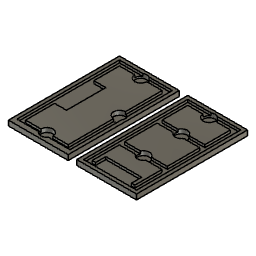
Circuit Template v1 v1 (Autodesk Fusion 360 design; units mm, degrees)
Autodesk Fusion 360 part; units mm, degrees
note: some values were not read from the file. Set by a fixed rule: which sketch regions a step uses.
sketch "Sketch1" plane through (0, 0, 0) normal (0, 0, 1) x (1, 0, 0)
  line L0 (0, 0) -> (88.9, 0)
  line L1 (88.9, 0) -> (88.9, 165.1)
  line L2 (88.9, 165.1) -> (0, 165.1)
  line L3 (0, 165.1) -> (0, 0)
  constraint horizontal L0
  constraint vertical L1
  constraint horizontal L2
  constraint vertical L3
  constraint coincident L0.start L3.end
extrude "Extrude1" add sketch "Sketch1" along normal blind 7.62 makes body 1
sketch "Sketch2" plane through (0, 0, 7.62) normal (0, 0, 1) x (-1, 0, 0)
  line L0 (0, -165.1) -> (0, 0)
  line L1 (0, 0) -> (-88.9, 0)
  line L2 (-88.9, 0) -> (-88.9, -165.1)
  line L3 (-88.9, -165.1) -> (0, -165.1)
  line L4 (-5.08, -7.62) -> (-83.82, -7.62)
  line L5 (-83.82, -7.62) -> (-83.82, -160.02)
  line L6 (-83.82, -160.02) -> (-5.08, -160.02)
  line L7 (-5.08, -160.02) -> (-5.08, -7.62)
  line L8 (-12.7, -152.4) -> (-76.2, -152.4)
  line L9 (-76.2, -152.4) -> (-76.2, -12.7)
  line L10 (-76.2, -12.7) -> (-12.7, -12.7)
  line L11 (-12.7, -12.7) -> (-12.7, -152.4)
  constraint horizontal L4
  constraint vertical L5
  constraint horizontal L6
  constraint vertical L7
  constraint horizontal L8
  constraint vertical L9
  constraint horizontal L10
  constraint vertical L11
copy_body "CopyPasteBodies1" bodies 1 makes body 2
move_body "Move1" bodies 2 to x (1, 0, 0) y (0, 1, 0) z (0, 0, 1) at (101.6, 0, 0)
sketch "Sketch3" plane through (0, 0, 7.62) normal (0, 0, 1) x (1, 0, 0)
  line L0 (5.08, 55.88) -> (30.48, 55.88)
  line L1 (30.48, 55.88) -> (30.48, 114.3)
  line L2 (30.48, 114.3) -> (5.08, 114.3)
  line L3 (5.08, 114.3) -> (5.08, 55.88)
  circle A0 centre (43.18, 10.16) radius 7.62
  circle A1 centre (78.74, 76.2) radius 7.62
  circle A2 centre (45.72, 154.94) radius 7.62
  dimension "d3" = 15.24
  dimension "d4" = 15.24
  constraint horizontal L0
  constraint vertical L1
  constraint horizontal L2
  constraint vertical L3
  measures "d3" diameter of A1
  measures "d4" diameter of A2
extrude "Extrude2" cut sketch "Sketch3" against normal blind 3.81 contours L0 L1 L2 L3 bodies 1
extrude "Extrude3" cut sketch "Sketch2" against normal blind 3.81 contours L4 L5 L6 L7 bodies 1
sketch "Sketch4" plane through (0, 0, 7.62) normal (0, 0, 1) x (-1, 0, 0)
  line L0 (-12.7, -55.88) -> (-12.7, -12.7)
  line L1 (-12.7, -12.7) -> (-76.2, -12.7)
  line L2 (-76.2, -12.7) -> (-76.2, -152.4)
  line L3 (-76.2, -152.4) -> (-12.7, -152.4)
  line L4 (-12.7, -152.4) -> (-12.7, -114.3)
  line L5 (-12.7, -114.3) -> (-30.48, -114.3)
  line L6 (-30.48, -114.3) -> (-30.48, -55.88)
  line L7 (-30.48, -55.88) -> (-12.7, -55.88)
  circle A0 centre (-44.45, -12.7) radius 8.89
  circle A1 centre (-76.2, -88.9) radius 8.89
  circle A2 centre (-44.45, -152.4) radius 8.89
  dimension "d10" = 17.78
  dimension "d11" = 17.78
  dimension "d12" = 17.78
  constraint midpoint L1 A0.centre
  constraint coincident L2 A1.centre
  constraint midpoint L3 A2.centre
  measures "d10" diameter of A0
  measures "d11" diameter of A1
  measures "d12" diameter of A2
extrude "Extrude4" cut sketch "Sketch4" against normal blind 6.35 contours L1 A0 picked at (-42.6024, -16.7637) bodies 1
extrude "Extrude5" cut sketch "Sketch4" against normal blind 6.35 contours L1 A0 picked at (-47.2515, -10.5408) bodies 1
extrude "Extrude6" cut sketch "Sketch4" against normal blind 6.35 contours L2 A1 | L2 A1 bodies 1
extrude "Extrude7" cut sketch "Sketch4" against normal blind 6.35 contours L3 A2 | L3 A2 bodies 1
sketch "Sketch5" plane through (0, 0, 7.62) normal (0, 0, 1) x (-1, 0, 0)
  line L0 (-101.6, -165.1) -> (-101.6, 0)
  line L1 (-101.6, 0) -> (-190.5, 0)
  line L2 (-190.5, 0) -> (-190.5, -165.1)
  line L3 (-190.5, -165.1) -> (-101.6, -165.1)
  line L4 (-106.68, -160.02) -> (-185.42, -160.02)
  line L5 (-185.42, -160.02) -> (-185.42, -5.08)
  line L6 (-185.42, -5.08) -> (-106.68, -5.08)
  line L7 (-106.68, -5.08) -> (-106.68, -160.02)
  line L8 (-177.8, -10.16) -> (-114.3, -10.16)
  line L9 (-114.3, -10.16) -> (-114.3, -152.4)
  line L10 (-114.3, -152.4) -> (-177.8, -152.4)
  line L11 (-177.8, -152.4) -> (-177.8, -10.16)
  line L12 (-114.3, -50.5992) -> (-177.8, -50.5992)
  line L13 (-177.8, -50.5992) -> (-177.8, -58.42)
  line L14 (-177.8, -58.42) -> (-114.3, -58.42)
  line L15 (-114.3, -58.42) -> (-114.3, -50.5992)
  line L16 (-177.8, -106.68) -> (-114.3, -106.68)
  line L17 (-114.3, -106.68) -> (-114.3, -114.3)
  line L18 (-114.3, -114.3) -> (-177.8, -114.3)
  line L19 (-177.8, -114.3) -> (-177.8, -106.68)
  circle A0 centre (-146.05, -152.4) radius 8.89
  circle A1 centre (-146.05, -110.9548) radius 8.89
  circle A2 centre (-146.05, -54.7727) radius 8.89
  line L20 (-134.62, -5.08) -> (-167.64, -5.08)
  line L21 (-167.64, -5.08) -> (-167.64, -25.4)
  line L22 (-167.64, -25.4) -> (-134.62, -25.4)
  line L23 (-134.62, -25.4) -> (-134.62, -5.08)
  line L24 (-134.62, -25.4) -> (-127, -25.4)
  line L25 (-127, -25.4) -> (-127, -5.08)
  line L26 (-127, -5.08) -> (-134.62, -5.08)
  line L27 (-134.62, -5.08) -> (-134.62, -25.4)
  line L28 (-127, -25.4) -> (-119.38, -25.4)
  line L29 (-119.38, -25.4) -> (-119.38, -5.08)
  line L30 (-119.38, -5.08) -> (-127, -5.08)
  line L31 (-127, -5.08) -> (-127, -25.4)
  line L32 (-167.64, -25.4) -> (-172.72, -25.4)
  line L33 (-172.72, -25.4) -> (-172.72, -5.08)
  line L34 (-172.72, -5.08) -> (-167.64, -5.08)
  line L35 (-167.64, -5.08) -> (-167.64, -25.4)
  dimension "d21" = 17.78
  dimension "d22" = 17.78
  dimension "d23" = 17.78
  constraint horizontal L4
  constraint vertical L5
  constraint horizontal L6
  constraint vertical L7
  constraint horizontal L8
  constraint vertical L9
  constraint horizontal L10
  constraint vertical L11
  constraint horizontal L12
  constraint vertical L13
  constraint horizontal L14
  constraint vertical L15
  constraint coincident L11 L13.end
  constraint coincident L9 L12.start
  constraint horizontal L16
  constraint vertical L17
  constraint horizontal L18
  constraint vertical L19
  constraint coincident L9 L17.end
  constraint coincident L11 L16.start
  constraint midpoint L10 A0.centre
  constraint horizontal L20
  constraint vertical L21
  constraint horizontal L22
  constraint vertical L23
  constraint coincident L6 L20.start
  constraint horizontal L24
  constraint vertical L25
  constraint horizontal L26
  constraint vertical L27
  constraint coincident L6 L25.end
  constraint horizontal L28
  constraint vertical L29
  constraint horizontal L30
  constraint vertical L31
  constraint coincident L6 L29.end
  constraint horizontal L32
  constraint vertical L33
  constraint horizontal L34
  constraint vertical L35
  constraint coincident L6 L33.end
  measures "d21" diameter of A0
  measures "d22" diameter of A1
  measures "d23" diameter of A2
extrude "Extrude8" cut sketch "Sketch5" against normal blind 3.81 contours L6 L8 L25 L29 L30 L31 | L6 L8 L23 L25 L26 L27 L31 | L8 L25 L28 L29 L31 | L6 L8 L20 L21 L23 L27 L35 | L8 L23 L24 L25 L27 L31 | L6 L8 L21 L33 L34 L35 | L8 L21 L22 L23 L27 L35 | L8 L21 L32 L33 L35 bodies 2
extrude "Extrude9" cut sketch "Sketch5" against normal blind 3.81 contours L4 L6 L7 L8 L9 L10 L15 L17 A0 L29 | L4 L5 L6 L8 L10 L11 L13 L19 A0 L33 | L9 L16 L17 L18 A1 | L11 L16 L18 L19 A1 | L9 L12 L14 L15 A2 | L11 L12 L13 L14 A2 bodies 2
extrude "Extrude10" cut sketch "Sketch5" against normal blind 6.35 contours L4 A0 | L4 L10 A0 | L10 A0 | L18 A1 | L16 L18 A1 | L16 A1 | L12 L14 A2 | L12 A2 | L14 A2 bodies 2
